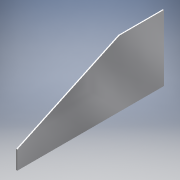
# Autodesk Inventor part: stay
Saved by Autodesk Inventor 2018.1 (Build 221171000, 171)
## iProperties
Created: 2017-10-18
Part Number: stay
Material: アルミニウム 6061
Document SubType Name: Modeling
Designer: kuwano
Density: 2.7 g/cm^3
Appearance: アルミニウム - フラット
Mass: 436.419 g
Surface Area: 1109.34 cm^2
Volume: 161.637 cm^3
Author: kuwano
Autodesk Inventor part; units mm, degrees
ref_plane "YZ Plane" through (0, 0, 0) normal (1, 0, 0) x (0, 1, 0)
ref_plane "XZ Plane" through (0, 0, 0) normal (0, 1, 0) x (-1, 0, 0)
ref_plane "XY Plane" through (0, 0, 0) normal (0, 0, 1) x (1, 0, 0)
sketch "スケッチ1" plane through (0, 0, 0) normal (1, 0, 0) x (0, 1, 0)
  line L0 (-40, 200) -> (-90, 200)
  line L1 (-90, 200) -> (-90, -200)
  line L2 (-90, -200) -> (90, -200)
  line L3 (90, -200) -> (90, -78.7859)
  line L4 (90, -78.7859) -> (-40, 200)
  line L5 (-126, 0) -> (126, 0) projected
  line L6 (0, -280) -> (0, 280) projected
  point P0 (0, 0)
  point P1 (-90, 0)
  point P2 (0, -200)
  dimension "d0" = 400
  dimension "d1" = 50
  dimension "d2" = 180
  dimension "d3" = 25
  constraints: 10 end point, 3 perpendicular, 2 midpoint, 2 point on line, 1 horizontal
  measures "d0" distance of L0.end L1.end
  measures "d1" distance of L0.start L0.end
  measures "d2" distance of L1.end L2.end
  measures "d3" angle of L1 L4
extrude "押し出し1" add sketch "スケッチ1" along normal blind 3
